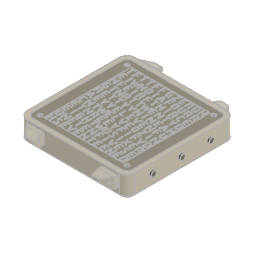
Wordy Watch v19 (Autodesk Fusion 360 design; units mm, degrees)
Autodesk Fusion 360 part; units mm, degrees
(part 1 of 4)
sketch "BatteryProfile" plane through (0, 0, 0) normal (0, 1, 0) x (1, 0, 0) in component "LiPo Battery"
  line L0 (-8.25, -1.75) -> (8.25, -1.75)
  line L1 (0, 0) -> (0, -1.75) construction
  line L2 (0, 0) -> (1, 0) construction
  line L3 (-8.25, 1.75) -> (8.25, 1.75)
  arc A0 (-8.25, 1.75) -> (-8.25, -1.75) centre (-8.25, 0) ccw
  arc A1 (8.25, -1.75) -> (8.25, 1.75) centre (8.25, 0) ccw
  line L4 (8.25, -1.75) -> (8.25, 1.75) construction
  line L5 (-8.25, -1.75) -> (-8.25, 1.75) construction
  point P0 (0, -1.75)
  dimension "d4" = 16.5
  dimension "d7" = 1.75
  dimension "d8" = 1
  constraint horizontal L0
  constraint coincident L1.start L2.start
  constraint vertical L1
  constraint midpoint L0 P0
  constraint coincident P0 L1.end
  constraint perpendicular L1 L2
  constraint symmetric L0.start L2 L3.start
  constraint symmetric L0.end L2 L3.end
  constraint coincident A1.centre L4
  constraint coincident A0.centre L5
  measures "d4" distance of L0.start L0.end
  measures "d7" distance of L1.start P0
  measures "d8" distance of L1.start L2.end
extrude "Extrude1" add sketch "BatteryProfile" along normal blind 25 makes body 1 in component "LiPo Battery"
sketch "PCBTop" plane through (0, 0, 0) normal (0, 0, 1) x (1, 0, 0) in component "PCB"
  line L0 (18, -18) -> (-18, -18)
  line L1 (-18, -18) -> (-18, 18)
  line L2 (-18, 18) -> (18, 18)
  line L3 (18, 18) -> (18, -18)
  line L4 (18, -18) -> (-18, 18) construction
  line L5 (-18, -18) -> (18, 18) construction
  line L6 (-9, -7.5) -> (-17, -7.5)
  line L7 (-17, -7.5) -> (-17, -13)
  line L8 (-17, -13) -> (-9, -13)
  line L9 (-9, -13) -> (-9, -7.5)
  line L10 (-9, -7.5) -> (-17, -13) construction
  line L11 (-17, -7.5) -> (-9, -13) construction
  line L12 (17.5, 8.6) -> (14.5, 8.6)
  line L13 (14.5, 8.6) -> (14.5, 13.4)
  line L14 (14.5, 13.4) -> (17.5, 13.4)
  line L15 (17.5, 13.4) -> (17.5, 8.6)
  line L16 (17.5, 8.6) -> (14.5, 13.4) construction
  line L17 (14.5, 8.6) -> (17.5, 13.4) construction
  line L18 (17.5, -2.4) -> (14.5, -2.4)
  line L19 (14.5, -2.4) -> (14.5, 2.4)
  line L20 (14.5, 2.4) -> (17.5, 2.4)
  line L21 (17.5, 2.4) -> (17.5, -2.4)
  line L22 (17.5, -13.4) -> (14.5, -13.4)
  line L23 (14.5, -13.4) -> (14.5, -8.6)
  line L24 (14.5, -8.6) -> (17.5, -8.6)
  line L25 (17.5, -8.6) -> (17.5, -13.4)
  line L26 (16.5, -16.5) -> (-16.5, -16.5) construction
  line L27 (-16.5, -16.5) -> (-16.5, 16.5) construction
  line L28 (-16.5, 16.5) -> (16.5, 16.5) construction
  line L29 (16.5, 16.5) -> (16.5, -16.5) construction
  line L30 (16.5, -16.5) -> (-16.5, 16.5) construction
  line L31 (-16.5, -16.5) -> (16.5, 16.5) construction
  circle A0 centre (-16.5, 16.5) radius 0.8
  circle A1 centre (16.5, 16.5) radius 0.8
  circle A2 centre (16.5, -16.5) radius 0.8
  circle A3 centre (-16.5, -16.5) radius 0.8
  point P0 (-13, -10.25)
  point P1 (16, 11)
  dimension "d79" = 36
  dimension "d80" = 36
  dimension "d83" = 8
  dimension "d84" = 5.5
  dimension "d85" = 5
  dimension "d87" = 3
  dimension "d88" = 4.8
  dimension "d89" = 2
  dimension "d90" = 7
  dimension "d93" = 11
  dimension "d94" = -22
  dimension "d178" = 33
  dimension "d179" = 33
  dimension "d180" = 1.6
  dimension "d181" = 1.6
  dimension "d182" = 1.6
  dimension "d183" = 1.6
  dimension "d239" = 7.75
  constraint horizontal L0
  constraint perpendicular L0 L1
  constraint parallel L0 L2
  constraint parallel L1 L3
  constraint coincident L4 origin
  constraint coincident L5 origin
  constraint horizontal L6
  constraint perpendicular L6 L7
  constraint parallel L6 L8
  constraint parallel L7 L9
  constraint coincident L10 P0
  constraint coincident L11 P0
  constraint horizontal L12
  constraint perpendicular L12 L13
  constraint parallel L12 L14
  constraint parallel L13 L15
  constraint coincident L16 P1
  constraint coincident L17 P1
  constraint horizontal L26
  constraint perpendicular L26 L27
  constraint parallel L26 L28
  constraint parallel L27 L29
  constraint coincident L30 origin
  constraint coincident L31 origin
  constraint coincident L27.end L28.start
  constraint coincident L28.end L29.start
  constraint coincident L26.start L29.end
  constraint coincident L26.end L27.start
  measures "d79" distance of L1.end L2.end
  measures "d80" distance of L0.end L1.end
  measures "d83" distance of L7.end L8.end
  measures "d84" distance of L6.end L7.end
  measures "d85" distance of L1 P0
  measures "d87" distance of L13.end L14.end
  measures "d88" distance of L12.end L13.end
  measures "d89" distance of L3 P1
  measures "d90" distance of L2 P1
  measures "d178" distance of L27.end L28.end
  measures "d179" distance of L26.end L27.end
  measures "d180" diameter of A0
  measures "d181" diameter of A1
  measures "d182" diameter of A2
  measures "d183" diameter of A3
  measures "d239" distance of L0 P0
sketch "USBC" plane through (0, 0, 0) normal (1, 0, 0) x (0, 1, 0) in component "PCB"
  line L0 (-18, 0) -> (18, 0)
  line L1 (4.1, 1) -> (9.9, 1)
  line L2 (9.9, 1) -> (9.9, 3.7)
  line L3 (9.9, 3.7) -> (4.1, 3.7)
  line L4 (4.1, 3.7) -> (4.1, 1)
  line L5 (4.1, 1) -> (9.9, 3.7) construction
  line L6 (9.9, 1) -> (4.1, 3.7) construction
  arc A0 (4.1, 3.7) -> (4.1, 1) centre (4.1, 2.35) ccw
  arc A1 (9.9, 1) -> (9.9, 3.7) centre (9.9, 2.35) ccw
  line L7 (7, 1) -> (7, 0) construction
  line L8 (4.1, 1) -> (4.1, 0)
  line L9 (9.9, 1) -> (9.9, 0)
  line L10 (9.9, 0) -> (4.1, 0)
  point P0 (7, 2.35)
  point P1 (7, 3.7)
  point P2 (18, 0)
  dimension "d95" = 5.8
  dimension "d96" = 2.7
  dimension "d103" = 1
  dimension "d238" = 11
  constraint horizontal L1
  constraint perpendicular L1 L2
  constraint parallel L1 L3
  constraint parallel L2 L4
  constraint coincident L5 P0
  constraint coincident L6 P0
  constraint midpoint L4 A0.centre
  constraint midpoint L2 A1.centre
  constraint midpoint L3 P1
  constraint midpoint L1 L7.start
  constraint coincident L0 L7.end
  constraint perpendicular L0 L7
  constraint coincident L0 L8.end
  constraint perpendicular L0 L8
  constraint coincident L0 L9.end
  constraint perpendicular L0 L9
  measures "d95" distance of L2.end L3.end
  measures "d96" distance of L1.end L2.end
  measures "d103" distance of L0 L1
  measures "d238" distance of L7.end P2
extrude "Extrude1'" add sketch "PCBTop" along normal blind 0.8 separate body contours L0 L1 L2 L3 | L6 L7 L8 L9 | L12 L13 L14 L15 | L18 L19 L20 L21 | L22 L23 L24 L25 makes body 2 in component "PCB"
extrude "Extrude2" add sketch "PCBTop" along normal blind 2.8 contours L12 L13 L14 L15 | L18 L19 L20 L21 | L22 L23 L24 L25 bodies 2 in component "PCB"
extrude "Extrude3" add sketch "PCBTop" along normal blind 3.8 contours L6 L7 L8 L9 bodies 2 in component "PCB"
extrude "Extrude4" add sketch "USBC" along normal blind 7 and the other way blind 1 from surface at -18 bodies 2 in component "PCB"
fillet "Fillet1" radius 2 4 edges at (-18, -18, 0.4) (18, -18, 0.4) (18, 18, 0.4) (-18, 18, 0.4) on bodies 2 in component "PCB"
sketch "ButtonBack" plane through (0, 0, 0) normal (0, 0, 1) x (1, 0, 0) in component "Case Button"
  line L0 (1.1, -0.55) -> (-1.1, -0.55)
  line L1 (-1.1, -0.55) -> (-1.1, 0.55)
  line L2 (-1.1, 0.55) -> (1.1, 0.55)
  line L3 (1.1, 0.55) -> (1.1, -0.55)
  line L4 (1.1, -0.55) -> (-1.1, 0.55) construction
  line L5 (-1.1, -0.55) -> (1.1, 0.55) construction
  circle A0 centre (0, 0) radius 1.75
  line L6 (-1.1, 0.55) -> (-1.1, 1.3611)
  line L7 (1.1, 0.55) -> (1.1, 1.3611)
  dimension "d202" = 1.1
  dimension "d203" = 2.2
  dimension "d204" = 3.5
  constraint horizontal L0
  constraint perpendicular L0 L1
  constraint parallel L0 L2
  constraint parallel L1 L3
  constraint coincident L4 A0.centre
  constraint coincident L5 A0.centre
  constraint coincident A0.centre origin
  constraint coincident A0 L6.end
  constraint perpendicular L2 L6
  constraint coincident A0 L7.end
  constraint perpendicular L2 L7
  measures "d202" distance of L0.end L1.end
  measures "d203" distance of L1.end L2.end
  measures "d204" diameter of A0
sketch "ButtonFront" plane through (0, 0, 0) normal (0, 0, 1) x (1, 0, 0) in component "Case Button"
  circle A0 centre (0, 0) radius 1
  dimension "d205" = 2
  constraint coincident A0.centre origin
  measures "d205" diameter of A0
extrude "Extrude1''" add sketch "ButtonBack" along normal blind 0.5 separate body contours L0 L1 L3 A0 L6 L7 makes body 3 in component "Case Button"
extrude "Extrude2'" add sketch "ButtonBack" along normal blind 0.5 from surface at 0.5 bodies 3 in component "Case Button"
extrude "Extrude3'" add sketch "ButtonFront" along normal blind 1.6 from surface at 1 bodies 3 in component "Case Button"
pattern_linear "R-Pattern1" count 3 spacing 11 along (1, 0, 0) of bodies 3 makes body 4 at (11.9988, -0.0498, 2.0667) makes body 5 at (22.9988, -0.0498, 2.0667) in component "Case Button"
sketch "CaseOuter" plane through (0, 0, 0) normal (0, 0, 1) x (1, 0, 0) in component "WatchCase"
  line L0 (-20.5, 20.5) -> (20.5, 20.5)
  line L1 (20.5, 20.5) -> (20.5, -20.5)
  line L2 (20.5, -20.5) -> (-20.5, -20.5)
  line L3 (-20.5, -20.5) -> (-20.5, 20.5)
  line L4 (-20.5, 20.5) -> (20.5, -20.5) construction
  line L5 (20.5, 20.5) -> (-20.5, -20.5) construction
  line L6 (-18.9, -18.9) -> (-18.9, 18.9)
  line L7 (-18.9, 18.9) -> (18.9, 18.9)
  line L8 (18.9, 18.9) -> (18.9, -18.9)
  line L9 (18.9, -18.9) -> (-18.9, -18.9)
  dimension "d42" = 41
  dimension "d43" = 41
  dimension "d44" = 1.6
  constraint horizontal L0
  constraint perpendicular L0 L1
  constraint parallel L0 L2
  constraint parallel L1 L3
  constraint coincident L4 origin
  constraint coincident L5 origin
  measures "d42" distance of L1.end L2.end
  measures "d43" distance of L0.end L1.end
sketch "CaseFixing" plane through (0, 0, 0) normal (0, 0, 1) x (1, 0, 0) in component "WatchCase"
  line L0 (16.5, -16.5) -> (-16.5, -16.5) construction
  line L1 (-16.5, -16.5) -> (-16.5, 16.5) construction
  line L2 (-16.5, 16.5) -> (16.5, 16.5) construction
  line L3 (16.5, 16.5) -> (16.5, -16.5) construction
  line L4 (16.5, -16.5) -> (-16.5, 16.5) construction
  line L5 (-16.5, -16.5) -> (16.5, 16.5) construction
  circle A0 centre (-16.5, 16.5) radius 0.6
  circle A1 centre (16.5, 16.5) radius 0.6
  circle A2 centre (-16.5, -16.5) radius 0.6
  circle A3 centre (16.5, -16.5) radius 0.6
  dimension "d32" = 33
  dimension "d33" = 33
  dimension "d34" = 1.2
  dimension "d35" = 1.2
  dimension "d36" = 1.2
  dimension "d37" = 1.2
  constraint horizontal L0
  constraint perpendicular L0 L1
  constraint parallel L0 L2
  constraint parallel L1 L3
  constraint coincident L4 origin
  constraint coincident L5 origin
  constraint coincident L1.end L2.start
  constraint coincident L2.end L3.start
  constraint coincident L0.end L1.start
  constraint coincident L0.start L3.end
  measures "d32" distance of L0.end L1.end
  measures "d33" distance of L1.end L2.end
  measures "d34" diameter of A0
  measures "d35" diameter of A1
  measures "d36" diameter of A2
  measures "d37" diameter of A3
sketch "CaseFixingBoss" plane through (0, 0, 0) normal (0, 0, 1) x (1, 0, 0) in component "WatchCase"
  line L0 (16.5, 16.5) -> (16.5, -16.5) construction
  circle A0 centre (-16.5, 16.5) radius 2.3
  circle A1 centre (16.5, 16.5) radius 2.3
  circle A2 centre (-16.5, -16.5) radius 2.3
  circle A3 centre (16.5, -16.5) radius 2.3
  line L1 (-16.5, 16.5) -> (16.5, 16.5) construction
  line L2 (-16.5, -16.5) -> (-16.5, 16.5) construction
  line L3 (16.5, -16.5) -> (-16.5, -16.5) construction
  dimension "d38" = 4.6
  dimension "d39" = 4.6
  dimension "d40" = 4.6
  dimension "d41" = 4.6
  constraint coincident A0.centre L1.start
  constraint coincident L0.start A1.centre
  constraint coincident A2.centre L2.start
  constraint coincident L0.end A3.centre
  measures "d38" diameter of A0
  measures "d39" diameter of A1
  measures "d40" diameter of A2
  measures "d41" diameter of A3
extrude "Extrude1'''" add sketch "CaseOuter" along normal blind 1.3 separate body contours L0 L1 L2 L3 | L6 L7 L8 L9 makes body 6 in component "WatchCase"
sketch "CaseCorners" plane through (0, 0, 0) normal (0, 0, 1) x (1, 0, 0) in component "WatchCase"
  line L0 (-20.5, -20.5) -> (20.5, -20.5)
  line L1 (20.5, -20.5) -> (20.5, 20.5)
  line L2 (20.5, 20.5) -> (-20.5, 20.5)
  line L3 (-20.5, 20.5) -> (-20.5, -20.5)
  line L4 (-16.5, 16.5) -> (16.5, 16.5)
  line L5 (-16.5, -16.5) -> (-16.5, 16.5)
  line L6 (16.5, -16.5) -> (-16.5, -16.5)
  line L7 (16.5, 16.5) -> (16.5, -16.5)
  line L8 (-16.5, 16.5) -> (-16.5, 20.5)
  line L9 (-16.5, 16.5) -> (-20.5, 16.5)
  line L10 (16.5, 16.5) -> (16.5, 20.5)
  line L11 (16.5, 16.5) -> (20.5, 16.5)
  line L12 (16.5, -16.5) -> (16.5, -20.5)
  line L13 (16.5, -16.5) -> (20.5, -16.5)
  line L14 (-16.5, -16.5) -> (-16.5, -20.5)
  line L15 (-16.5, -16.5) -> (-20.5, -16.5)
  constraint coincident L4.start L5.end
  constraint coincident L2 L8.end
  constraint perpendicular L2 L8
  constraint coincident L3 L9.end
  constraint perpendicular L3 L9
  constraint coincident L4.end L7.start
  constraint coincident L2 L10.end
  constraint perpendicular L2 L10
  constraint coincident L1 L11.end
  constraint perpendicular L1 L11
  constraint coincident L6.start L7.end
  constraint coincident L0 L12.end
  constraint perpendicular L0 L12
  constraint coincident L1 L13.end
  constraint perpendicular L1 L13
  constraint coincident L5.start L6.end
  constraint coincident L0 L14.end
  constraint perpendicular L0 L14
  constraint coincident L3 L15.end
  constraint perpendicular L3 L15
extrude "Extrude2''" add sketch "CaseFixingBoss" along normal blind 4.5 from surface at 1.3 separate body makes body 7 at (18.7971, 16.3854, 4.3) makes body 8 at (18.7971, -16.6146, 4.3) makes body 9 at (-14.2029, 16.3854, 4.3) makes body 10 at (-14.2029, -16.6146, 4.3) in component "WatchCase"
extrude "Extrude3''" add sketch "CaseOuter" along normal blind 8.1 bodies 6 in component "WatchCase"
extrude "Extrude4'" add sketch "CaseCorners" along normal up to surface (5.8 mm away) contours L0 L3 L14 L15 | L0 L1 L12 L13 | L2 L3 L8 L9 | L1 L2 L10 L11 bodies 6 7 8 9 10 in component "WatchCase"
extrude "Extrude5" cut sketch "CaseFixing" along normal up to surface (4.8 mm away) from surface at 1 bodies 6 in component "WatchCase"
fillet "Fillet1'" radius 2 4 edges at (18.9, 18.9, 6.95) (-18.9, 18.9, 6.95) (18.9, -18.9, 6.95) (-18.9, -18.9, 6.95) on bodies 6 in component "WatchCase"
fillet "Fillet2" radius 3 4 edges at (20.5, -20.5, 4.05) (-20.5, -20.5, 4.05) (-20.5, 20.5, 4.05) (20.5, 20.5, 4.05) on bodies 6 in component "WatchCase"
chamfer "Chamfer1" distance 1 angle 45 8 edges at (0, -20.5, 0) (-19.6213, -19.6213, 0) (-20.5, 0, 0) (-19.6213, 19.6213, 0) (0, 20.5, 0) (19.6213, 19.6213, 0) (20.5, 0, 0) (19.6213, -19.6213, 0) on bodies 6 in component "WatchCase"
sketch "Strap Bracket" plane through (0, 0, 0) normal (0, 0, 1) x (1, 0, 0) in component "WatchCase"
  line L0 (17.5, 20.5) -> (-17.5, 20.5)
  line L1 (-17.5, -20.5) -> (17.5, -20.5)
  line L2 (-17, 24.5) -> (-11, 24.5)
  line L3 (-11, 24.5) -> (-11, 20.5)
  line L4 (-11, 20.5) -> (-17, 20.5)
  line L5 (-17, 20.5) -> (-17, 24.5)
  line L6 (11, 24.5) -> (17, 24.5)
  line L7 (17, 24.5) -> (17, 20.5)
  line L8 (17, 20.5) -> (11, 20.5)
  line L9 (11, 20.5) -> (11, 24.5)
  line L10 (17.5, 20.5) -> (17.5, -20.5) construction
  line L11 (17.5, 0) -> (12.5, 0) construction
  point P0 (0, 20.5)
  dimension "d149" = 6
  dimension "d150" = 4
  dimension "d151" = 6
  dimension "d152" = 4
  dimension "d153" = 11
  dimension "d154" = 11
  dimension "d155" = 5
  constraint horizontal L2
  constraint vertical L3
  constraint horizontal L4
  constraint vertical L5
  constraint midpoint L0 P0
  constraint coincident L0 L3.end
  constraint horizontal L6
  constraint vertical L7
  constraint horizontal L8
  constraint vertical L9
  constraint coincident L0 L8.end
  constraint coincident L0.start L10.start
  constraint coincident L1.end L10.end
  constraint midpoint L10 L11.start
  constraint perpendicular L10 L11
  measures "d149" distance of L2.start L2.end
  measures "d150" distance of L2.start L4.end
  measures "d151" distance of L6.start L6.end
  measures "d152" distance of L6.start L8.end
  measures "d153" distance of L3.end P0
  measures "d154" distance of P0 L8.end
  measures "d155" distance of L11.start L11.end
extrude "Extrude6" add sketch "Strap Bracket" against normal blind 4 from surface at 7.1 separate body makes body 11 at (-13, 20.5, 4.4333) makes body 12 at (13, 24.5, 5.7667) in component "WatchCase"
sketch "BracketProfile" plane through (17, 0, 0) normal (1, 0, 0) x (0, 1, 0) in component "WatchCase"
  line L0 (24.5, 7.1) -> (20.5, 7.1)
  line L1 (20.5, 3.1) -> (24.5, 3.1)
  line L2 (24.5, 3.1) -> (24.5, 7.1)
  line L3 (20.5, 7.1) -> (24.5, 3.1) construction
  circle A0 centre (22.5, 5.1) radius 0.5
  line L4 (20.5, 7.1) -> (20.5, 3.1)
  dimension "d162" = 1
  constraint coincident L0.end L3.start
  constraint coincident L1.end L2.start
  constraint midpoint L3 A0.centre
  measures "d162" diameter of A0
extrude "Extrude7" cut sketch "BracketProfile" against normal blind 10 from surface at -28 contours A0 bodies 12 6 11 in component "WatchCase"
extrude "Extrude8" cut sketch "BracketProfile" along normal blind 10 from surface at -6 contours A0 bodies 12 11 6 in component "WatchCase"
chamfer "Chamfer2" distance 1 angle 70 2 edges at (14, 24.5, 7.1) (-14, 24.5, 7.1) measured on face at (13, 24.5, 5.7667) measured on face at (-15, 24.5, 5.7667) on bodies 11 12 in component "WatchCase"
chamfer "Chamfer3" distance 2 angle 45 2 edges at (14, 24.5, 3.1) (-14, 24.5, 3.1) measured on face at (13, 23.1667, 3.1) measured on face at (-13, 21.8333, 3.1) on bodies 11 12 in component "WatchCase"
chamfer "Chamfer4" distance 3 angle 45 2 edges at (17, 24.5, 5.6) (-17, 24.5, 5.6) measured on face at (13, 24.5, 5.7667) measured on face at (-17, 21, 5.1) on bodies 11 12 in component "WatchCase"
mirror "Mirror1" about plane through (0, 0, 0) normal (0, 1, 0) of bodies 12 11 makes body 13 at (-13, -20.5, 4.4333) makes body 14 at (15, -20.5, 5.7667) in component "WatchCase"
combine "Combine1" operation add target body 6 tool bodies 11 12 14 13 in component "WatchCase"
sketch "USBC (2)" plane through (-20.5, 0, 0) normal (-1, 0, 0) x (0, -1, 0) in component "WatchCase"
  line L0 (-17.5, 1) -> (17.5, 1)
  line L1 (17.5, 1) -> (17.5, 8.1)
  line L2 (17.5, 8.1) -> (-17.5, 8.1)
  line L3 (-17.5, 8.1) -> (-17.5, 1)
  line L4 (4.1, 2.9) -> (9.9, 2.9)
  arc A0 (9.9, 2.9) -> (9.9, 5.6) centre (9.9, 4.25) ccw
  line L5 (9.9, 5.6) -> (9.9, 6.6)
  line L6 (9.9, 6.6) -> (4.1, 6.6)
  line L7 (4.1, 6.6) -> (4.1, 5.6)
  arc A1 (4.1, 5.6) -> (4.1, 2.9) centre (4.1, 4.25) ccw
  line L8 (10.1, 6.8) -> (3.9, 6.8)
  line L9 (3.9, 6.8) -> (3.9, 5.787)
  arc A2 (3.9, 5.787) -> (4.1, 2.7) centre (4.1, 4.25) ccw
  line L10 (4.1, 2.7) -> (9.9, 2.7)
  arc A3 (9.9, 2.7) -> (10.1, 5.787) centre (9.9, 4.25) ccw
  line L11 (10.1, 5.787) -> (10.1, 6.8)
  line L12 (3.9, 5.787) -> (10.1, 5.787)
  dimension "d184" = 0.2
extrude "Extrude9" cut sketch "USBC (2)" against normal up to surface (1.6 mm away) contours L4 A0 L5 L7 A1 L12 | L4 A0 L5 L7 A1 A2 L10 A3 L12 bodies 6 in component "WatchCase"
extrude "Extrude5'" cut sketch "USBC (2)" against normal up to surface (1.6 mm away) contours L4 A0 L5 L7 A1 L12 | L4 A0 L5 L7 A1 A2 L10 A3 L12 sketch seen with x (1, 0, 0) y (0, -1, 0) z (0, 0, -1) at (0, 0, 6.6) bodies 2 in component "PCB"
sketch "Buttons" plane through (20.5, 0, 0) normal (1, 0, 0) x (0, 1, 0) in component "WatchCase"
  line L0 (-17.5, 1) -> (17.5, 1)
  line L1 (17.5, 1) -> (17.5, 8.1)
  line L2 (17.5, 8.1) -> (-17.5, 8.1)
  line L3 (-17.5, 8.1) -> (-17.5, 1)
  line L4 (-8.6, 5.8) -> (-13.4, 5.8)
  line L5 (-13.4, 5.8) -> (-13.4, 3.8)
  line L6 (-13.4, 3.8) -> (-8.6, 3.8)
  line L7 (-8.6, 3.8) -> (-8.6, 5.8)
  line L8 (2.4, 5.8) -> (-2.4, 5.8)
  line L9 (-2.4, 5.8) -> (-2.4, 3.8)
  line L10 (-2.4, 3.8) -> (2.4, 3.8)
  line L11 (2.4, 3.8) -> (2.4, 5.8)
  line L12 (13.4, 5.8) -> (8.6, 5.8)
  line L13 (8.6, 5.8) -> (8.6, 3.8)
  line L14 (8.6, 3.8) -> (13.4, 3.8)
  line L15 (13.4, 3.8) -> (13.4, 5.8)
  line L16 (-13.4, 5.8) -> (-8.6, 3.8) construction
  line L17 (-10.04, 4.4) -> (-11.96, 4.4)
  line L18 (-11.96, 4.4) -> (-11.96, 5.2)
  line L19 (-11.96, 5.2) -> (-10.04, 5.2)
  line L20 (-10.04, 5.2) -> (-10.04, 4.4)
  line L21 (-10.04, 4.4) -> (-11.96, 5.2) construction
  line L22 (-11.96, 4.4) -> (-10.04, 5.2) construction
  line L23 (0.96, 5.2) -> (0.96, 4.4)
  line L24 (0.96, 4.4) -> (-0.96, 4.4)
  line L25 (-0.96, 5.2) -> (0.96, 5.2)
  line L26 (-0.96, 4.4) -> (-0.96, 5.2)
  line L27 (11.96, 5.2) -> (11.96, 4.4)
  line L28 (10.04, 5.2) -> (11.96, 5.2)
  line L29 (10.04, 4.4) -> (10.04, 5.2)
  line L30 (11.96, 4.4) -> (10.04, 4.4)
  line L31 (-2.4, 5.8) -> (2.4, 3.8) construction
  line L32 (8.6, 5.8) -> (13.4, 3.8) construction
  line L33 (0.96, 5.2) -> (-0.96, 4.4) construction
  line L34 (11.96, 5.2) -> (10.04, 4.4) construction
  point P0 (-11, 4.8)
  point P1 (11, 4.8)
  point P2 (11, 4.8)
  point P3 (0, 4.8)
  point P4 (0, 4.8)
  dimension "d189" = 1.92
  dimension "d190" = 0.8
  dimension "d191" = 1.92
  dimension "d192" = 0.8
  dimension "d193" = 1.92
  dimension "d194" = 0.8
  constraint coincident L4.end L5.start
  constraint coincident L6.end L7.start
  constraint horizontal L17
  constraint perpendicular L17 L18
  constraint parallel L17 L19
  constraint parallel L18 L20
  constraint coincident L21 P0
  constraint coincident L22 P0
  constraint midpoint L16 P0
  constraint horizontal L24
  constraint perpendicular L24 L26
  constraint parallel L24 L25
  constraint parallel L23 L26
  constraint horizontal L30
  constraint perpendicular L29 L30
  constraint parallel L28 L30
  constraint parallel L27 L29
  constraint coincident L8.end L9.start
  constraint coincident L10.end L11.start
  constraint coincident L12.end L13.start
  constraint coincident L14.end L15.start
  constraint midpoint L34 P2
  constraint midpoint L32 P2
  constraint coincident P2 P1
  constraint midpoint L33 P4
  constraint midpoint L31 P4
  constraint coincident P4 P3
  measures "d189" distance of L18.end L19.end
  measures "d190" distance of L17.end L18.end
  measures "d191" distance of L25.start L23.start
  measures "d192" distance of L24.end L25.start
  measures "d193" distance of L28.start L27.start
  measures "d194" distance of L29.start L28.start
sketch "ButtonHoles" plane through (20.5, 0, 0) normal (1, 0, 0) x (0, 1, 0) in component "WatchCase"
  circle A0 centre (-11, 4.8) radius 1.2
  circle A1 centre (0, 4.8) radius 1.2
  circle A2 centre (11, 4.8) radius 1.2
  circle A3 centre (-11, 4.8) radius 1.95
  circle A4 centre (0, 4.8) radius 1.95
  circle A5 centre (11, 4.8) radius 1.95
  point P0 (-11, 4.8)
  point P1 (0, 4.8)
  point P2 (11, 4.8)
  dimension "d215" = 2.4
  dimension "d216" = 2.4
  dimension "d218" = 2.4
  dimension "d219" = 3.9
  dimension "d220" = 3.9
  dimension "d221" = 3.9
  constraint coincident P0 A0.centre
  constraint coincident P1 A1.centre
  constraint coincident P2 A2.centre
  constraint concentric A2 A5
  measures "d215" diameter of A0
  measures "d216" diameter of A1
  measures "d218" diameter of A2
  measures "d219" diameter of A3
  measures "d220" diameter of A4
  measures "d221" diameter of A5
extrude "Extrude6'" [suppressed] in component "PCB"
extrude "Extrude10" cut sketch "ButtonHoles" along normal blind 0.7 from surface at -1.6 contours A0 | A1 | A2 | A3 | A4 | A5 bodies 6 in component "WatchCase"
extrude "Extrude11" cut sketch "ButtonHoles" against normal up to surface (1.6 mm away) contours A0 | A1 | A2 bodies 6 in component "WatchCase"
sketch "Sketch1" plane through (0, 0, 0) normal (0, 0, 1) x (1, 0, 0) in component "Watch Face Text"
  line L0 (30.097, -17.6641) -> (60.097, -17.6641)
  line L1 (60.097, -17.6641) -> (60.097, 15.3359)
  line L2 (60.097, 15.3359) -> (30.097, 15.3359)
  line L3 (30.097, 15.3359) -> (30.097, -17.6641)
  line L4 (31.1779, 14.8177) -> (30.5921, 14.8605)
  line L5 (30.5921, 14.8605) -> (30.5702, 14.9689)
  line L6 (30.5702, 14.9689) -> (30.727, 15.0359)
  line L7 (30.727, 15.0359) -> (32.0867, 15.0041)
  line L8 (32.0867, 15.0041) -> (32.1306, 14.898)
  line L9 (32.1306, 14.898) -> (31.967, 14.8177)
  line L10 (31.967, 14.8177) -> (31.5161, 14.8177)
  line L11 (31.5161, 14.8177) -> (31.4941, 12.6904)
  line L12 (31.4941, 12.6904) -> (31.2624, 12.65)
  line L13 (31.2624, 12.65) -> (31.1779, 12.745)
  line L14 (31.1779, 12.745) -> (31.1779, 14.8177)
  line L15 (3.0809, 34.4818) -> (3.0809, 34.4818)
  line L16 (33.4792, 13.945) -> (34.3317, 13.9132)
  line L17 (34.3317, 13.9132) -> (34.3755, 13.8071)
  line L18 (34.3755, 13.8071) -> (34.2119, 13.7268)
  line L19 (34.2119, 13.7268) -> (33.4792, 13.7268)
  line L20 (33.4792, 13.7268) -> (33.4573, 12.6904)
  line L21 (33.4573, 12.6904) -> (33.2256, 12.65)
  line L22 (33.2256, 12.65) -> (33.141, 12.745)
  line L23 (33.141, 12.745) -> (33.1629, 14.9814)
  line L24 (33.1629, 14.9814) -> (33.3101, 15.0359)
  line L25 (33.3101, 15.0359) -> (34.5036, 15.0041)
  line L26 (34.5036, 15.0041) -> (34.5474, 14.8989)
  line L27 (34.5474, 14.8989) -> (34.3838, 14.8177)
  line L28 (34.3838, 14.8177) -> (33.4792, 14.8177)
  line L29 (33.4792, 14.8177) -> (33.4792, 13.945)
  line L30 (5.3822, 33.6091) -> (5.3822, 33.6091)
  line L31 (36.1779, 14.8177) -> (35.5921, 14.8605)
  line L32 (35.5921, 14.8605) -> (35.5702, 14.9689)
  line L33 (35.5702, 14.9689) -> (35.727, 15.0359)
  line L34 (35.727, 15.0359) -> (37.0867, 15.0041)
  line L35 (37.0867, 15.0041) -> (37.1306, 14.898)
  line L36 (37.1306, 14.898) -> (36.967, 14.8177)
  line L37 (36.967, 14.8177) -> (36.5161, 14.8177)
  line L38 (36.5161, 14.8177) -> (36.4941, 12.6904)
  line L39 (36.4941, 12.6904) -> (36.2624, 12.65)
  line L40 (36.2624, 12.65) -> (36.1779, 12.745)
  line L41 (36.1779, 12.745) -> (36.1779, 14.8177)
  line L42 (8.0809, 34.4818) -> (8.0809, 34.4818)
  line L43 (38.6779, 14.8177) -> (38.0921, 14.8605)
  line L44 (38.0921, 14.8605) -> (38.0702, 14.9689)
  line L45 (38.0702, 14.9689) -> (38.227, 15.0359)
  line L46 (38.227, 15.0359) -> (39.5867, 15.0041)
  line L47 (39.5867, 15.0041) -> (39.6306, 14.898)
  line L48 (39.6306, 14.898) -> (39.467, 14.8177)
  line L49 (39.467, 14.8177) -> (39.0161, 14.8177)
  line L50 (39.0161, 14.8177) -> (38.9941, 12.6904)
  line L51 (38.9941, 12.6904) -> (38.7624, 12.65)
  line L52 (38.7624, 12.65) -> (38.6779, 12.745)
  line L53 (38.6779, 12.745) -> (38.6779, 14.8177)
  line L54 (10.5809, 34.4818) -> (10.5809, 34.4818)
  line L55 (40.9792, 13.945) -> (41.8317, 13.9132)
  line L56 (41.8317, 13.9132) -> (41.8755, 13.8071)
  line L57 (41.8755, 13.8071) -> (41.7119, 13.7268)
  line L58 (41.7119, 13.7268) -> (40.9792, 13.7268)
  line L59 (40.9792, 13.7268) -> (40.9573, 12.6904)
  line L60 (40.9573, 12.6904) -> (40.7256, 12.65)
  line L61 (40.7256, 12.65) -> (40.641, 12.745)
  line L62 (40.641, 12.745) -> (40.6629, 14.9814)
  line L63 (40.6629, 14.9814) -> (40.8101, 15.0359)
  line L64 (40.8101, 15.0359) -> (42.0036, 15.0041)
  line L65 (42.0036, 15.0041) -> (42.0474, 14.8989)
  line L66 (42.0474, 14.8989) -> (41.8838, 14.8177)
  line L67 (41.8838, 14.8177) -> (40.9792, 14.8177)
  line L68 (40.9792, 14.8177) -> (40.9792, 13.945)
  line L69 (12.8822, 33.6091) -> (12.8822, 33.6091)
  line L70 (43.4792, 13.945) -> (44.3317, 13.9132)
  line L71 (44.3317, 13.9132) -> (44.3755, 13.8071)
  line L72 (44.3755, 13.8071) -> (44.2119, 13.7268)
  line L73 (44.2119, 13.7268) -> (43.4792, 13.7268)
  line L74 (43.4792, 13.7268) -> (43.4573, 12.6904)
  line L75 (43.4573, 12.6904) -> (43.2256, 12.65)
  line L76 (43.2256, 12.65) -> (43.141, 12.745)
  line L77 (43.141, 12.745) -> (43.1629, 14.9814)
  line L78 (43.1629, 14.9814) -> (43.3101, 15.0359)
  line L79 (43.3101, 15.0359) -> (44.5036, 15.0041)
  line L80 (44.5036, 15.0041) -> (44.5474, 14.8989)
  line L81 (44.5474, 14.8989) -> (44.3838, 14.8177)
  line L82 (44.3838, 14.8177) -> (43.4792, 14.8177)
  line L83 (43.4792, 14.8177) -> (43.4792, 13.945)
  line L84 (15.3822, 33.6091) -> (15.3822, 33.6091)
  line L85 (46.9045, 14.882) -> (46.9463, 14.7785)
  line L86 (46.9463, 14.7785) -> (46.7415, 14.703)
  line L87 (46.7415, 14.703) -> (46.4641, 14.8096)
  line L88 (46.4641, 14.8096) -> (46.1753, 14.7983)
  line L89 (46.1753, 14.7983) -> (45.9927, 14.7062)
  line L90 (45.9927, 14.7062) -> (45.9175, 14.608)
  line L91 (45.9175, 14.608) -> (45.9067, 13.0986)
  line L92 (45.9067, 13.0986) -> (45.9604, 12.9946)
  line L93 (45.9604, 12.9946) -> (46.1244, 12.8881)
  line L94 (46.1244, 12.8881) -> (46.347, 12.8507)
  line L95 (46.347, 12.8507) -> (46.7908, 12.8507)
  line L96 (46.7908, 12.8507) -> (46.7908, 13.6739)
  line L97 (46.7908, 13.6739) -> (46.4795, 13.7288)
  line L98 (46.4795, 13.7288) -> (46.4795, 13.835)
  line L99 (46.4795, 13.835) -> (46.6244, 13.8887)
  line L100 (46.6244, 13.8887) -> (47.091, 13.8466)
  line L101 (47.091, 13.8466) -> (47.1237, 13.7813)
  line L102 (47.1237, 13.7813) -> (47.1021, 12.6908)
  line L103 (47.1021, 12.6908) -> (46.9573, 12.6359)
  line L104 (46.9573, 12.6359) -> (46.2423, 12.64)
  line L105 (46.2423, 12.64) -> (45.9598, 12.7007)
  line L106 (45.9598, 12.7007) -> (45.7282, 12.8321)
  line L107 (45.7282, 12.8321) -> (45.6271, 12.9431)
  line L108 (45.6271, 12.9431) -> (45.5766, 13.0677)
  line L109 (45.5766, 13.0677) -> (45.5766, 14.6023)
  line L110 (45.5766, 14.6023) -> (45.6271, 14.7272)
  line L111 (45.6271, 14.7272) -> (45.7282, 14.8385)
  line L112 (45.7282, 14.8385) -> (45.9598, 14.9707)
  line L113 (45.9598, 14.9707) -> (46.2423, 15.0318)
  line L114 (46.2423, 15.0318) -> (46.5519, 15.0188)
  line L115 (46.5519, 15.0188) -> (46.9045, 14.882)
  line L116 (18.8076, 34.5461) -> (18.8076, 34.5461)
  line L117 (49.2471, 14.8177) -> (48.079, 14.8495)
  line L118 (48.079, 14.8495) -> (48.0352, 14.9556)
  line L119 (48.0352, 14.9556) -> (48.1988, 15.0359)
  line L120 (48.1988, 15.0359) -> (49.6149, 15.0041)
  line L121 (49.6149, 15.0041) -> (49.653, 14.885)
  line L122 (49.653, 14.885) -> (48.4468, 12.8541)
  line L123 (48.4468, 12.8541) -> (49.6149, 12.8223)
  line L124 (49.6149, 12.8223) -> (49.6588, 12.7171)
  line L125 (49.6588, 12.7171) -> (49.4951, 12.6359)
  line L126 (49.4951, 12.6359) -> (48.0818, 12.6686)
  line L127 (48.0818, 12.6686) -> (48.0466, 12.7941)
  line L128 (48.0466, 12.7941) -> (49.2471, 14.8177)
  line L129 (21.1502, 34.4818) -> (21.1502, 34.4818)
  line L130 (50.641, 12.745) -> (50.6629, 14.9814)
  line L131 (50.6629, 14.9814) -> (50.8101, 15.0359)
  line L132 (50.8101, 15.0359) -> (52.0036, 15.0041)
  line L133 (52.0036, 15.0041) -> (52.0474, 14.8989)
  line L134 (52.0474, 14.8989) -> (51.8838, 14.8177)
  line L135 (51.8838, 14.8177) -> (50.9792, 14.8177)
  line L136 (50.9792, 14.8177) -> (50.9792, 13.945)
  line L137 (50.9792, 13.945) -> (51.8317, 13.9132)
  line L138 (51.8317, 13.9132) -> (51.8755, 13.8071)
  line L139 (51.8755, 13.8071) -> (51.7119, 13.7268)
  line L140 (51.7119, 13.7268) -> (50.9792, 13.7268)
  line L141 (50.9792, 13.7268) -> (50.9792, 12.8541)
  line L142 (50.9792, 12.8541) -> (52.0036, 12.8223)
  line L143 (52.0036, 12.8223) -> (52.0474, 12.7171)
  line L144 (52.0474, 12.7171) -> (51.8838, 12.6359)
  line L145 (51.8838, 12.6359) -> (50.6903, 12.6677)
  line L146 (50.6903, 12.6677) -> (50.641, 12.745)
  line L147 (22.544, 32.4091) -> (22.544, 32.4091)
  line L148 (53.9963, 13.625) -> (54.1977, 13.7268)
  line L149 (54.1977, 13.7268) -> (54.2415, 13.8359)
  line L150 (54.2415, 13.8359) -> (54.2304, 14.6571)
  line L151 (54.2304, 14.6571) -> (54.1071, 14.7735)
  line L152 (54.1071, 14.7735) -> (53.9033, 14.8177)
  line L153 (53.9033, 14.8177) -> (53.3397, 14.8177)
  line L154 (53.3397, 14.8177) -> (53.3178, 12.6904)
  line L155 (53.3178, 12.6904) -> (53.0861, 12.65)
  line L156 (53.0861, 12.65) -> (53.0015, 12.745)
  line L157 (53.0015, 12.745) -> (53.0234, 14.9814)
  line L158 (53.0234, 14.9814) -> (53.1706, 15.0359)
  line L159 (53.1706, 15.0359) -> (54.0804, 15.0217)
  line L160 (54.0804, 15.0217) -> (54.3126, 14.9469)
  line L161 (54.3126, 14.9469) -> (54.4914, 14.8165)
  line L162 (54.4914, 14.8165) -> (54.5576, 14.7138)
  line L163 (54.5576, 14.7138) -> (54.5797, 14.5995)
  line L164 (54.5797, 14.5995) -> (54.5742, 13.7774)
  line L165 (54.5742, 13.7774) -> (54.5304, 13.6691)
  line L166 (54.5304, 13.6691) -> (54.2528, 13.4614)
  line L167 (54.2528, 13.4614) -> (54.684, 12.7123)
  line L168 (54.684, 12.7123) -> (54.4726, 12.6395)
  line L169 (54.4726, 12.6395) -> (54.3711, 12.6959)
  line L170 (54.3711, 12.6959) -> (53.8709, 13.5343)
  line L171 (53.8709, 13.5343) -> (53.9963, 13.625)
  line L172 (25.8994, 33.2891) -> (25.8994, 33.2891)
  line L173 (56.6117, 14.827) -> (56.5159, 14.9251)
  line L174 (56.5159, 14.9251) -> (56.6403, 15.0306)
  line L175 (56.6403, 15.0306) -> (56.9045, 14.9505)
  line L176 (56.9045, 14.9505) -> (57.0328, 14.8443)
  line L177 (57.0328, 14.8443) -> (57.1098, 14.7244)
  line L178 (57.1098, 14.7244) -> (57.1355, 14.5908)
  line L179 (57.1355, 14.5908) -> (57.129, 13.0125)
  line L180 (57.129, 13.0125) -> (57.0777, 12.8857)
  line L181 (57.0777, 12.8857) -> (56.9751, 12.7727)
  line L182 (56.9751, 12.7727) -> (56.662, 12.6368)
  line L183 (56.662, 12.6368) -> (56.5173, 12.7307)
  line L184 (56.5173, 12.7307) -> (56.7644, 12.9697)
  line L185 (56.7644, 12.9697) -> (56.7975, 13.081)
  line L186 (56.7975, 13.081) -> (56.7939, 14.6298)
  line L187 (56.7939, 14.6298) -> (56.7387, 14.7353)
  line L188 (56.7387, 14.7353) -> (56.6117, 14.827)
  line L189 (28.5147, 34.4911) -> (28.5147, 34.4911)
  line L190 (55.9105, 15.0159) -> (56.1561, 14.9802)
  line L191 (56.1561, 14.9802) -> (56.1567, 14.8728)
  line L192 (56.1567, 14.8728) -> (55.9552, 14.7353)
  line L193 (55.9552, 14.7353) -> (55.9001, 14.6298)
  line L194 (55.9001, 14.6298) -> (55.9001, 13.042)
  line L195 (55.9001, 13.042) -> (55.9552, 12.9365)
  line L196 (55.9552, 12.9365) -> (56.1766, 12.7615)
  line L197 (56.1766, 12.7615) -> (56.0916, 12.6518)
  line L198 (56.0916, 12.6518) -> (55.7894, 12.7213)
  line L199 (55.7894, 12.7213) -> (55.6611, 12.8275)
  line L200 (55.6611, 12.8275) -> (55.5841, 12.9474)
  line L201 (55.5841, 12.9474) -> (55.5585, 13.081)
  line L202 (55.5585, 13.081) -> (55.5649, 14.6593)
  line L203 (55.5649, 14.6593) -> (55.6162, 14.7861)
  line L204 (55.6162, 14.7861) -> (55.7188, 14.8991)
  line L205 (55.7188, 14.8991) -> (55.9105, 15.0159)
  line L206 (27.8135, 34.68) -> (27.8135, 34.68)
  line L207 (58.0029, 12.745) -> (58.0248, 14.9814)
  line L208 (58.0248, 14.9814) -> (58.2566, 15.0218)
  line L209 (58.2566, 15.0218) -> (58.3411, 14.9268)
  line L210 (58.3411, 14.9268) -> (58.3411, 13.945)
  line L211 (58.3411, 13.945) -> (59.3528, 13.945)
  line L212 (59.3528, 13.945) -> (59.3747, 14.9814)
  line L213 (59.3747, 14.9814) -> (59.6065, 15.0218)
  line L214 (59.6065, 15.0218) -> (59.691, 14.9268)
  line L215 (59.691, 14.9268) -> (59.6691, 12.6904)
  line L216 (59.6691, 12.6904) -> (59.4374, 12.65)
  line L217 (59.4374, 12.65) -> (59.3528, 12.745)
  line L218 (59.3528, 12.745) -> (59.3528, 13.7268)
  line L219 (59.3528, 13.7268) -> (58.3411, 13.7268)
  line L220 (58.3411, 13.7268) -> (58.3192, 12.6904)
  line L221 (58.3192, 12.6904) -> (58.0875, 12.65)
  line L222 (58.0875, 12.65) -> (58.0029, 12.745)
  line L223 (29.906, 32.4091) -> (29.906, 32.4091)
  line L224 (30.641, 9.745) -> (30.6629, 11.9814)
  line L225 (30.6629, 11.9814) -> (30.8101, 12.0359)
  line L226 (30.8101, 12.0359) -> (32.0036, 12.0041)
  line L227 (32.0036, 12.0041) -> (32.0474, 11.8989)
  line L228 (32.0474, 11.8989) -> (31.8838, 11.8177)
  line L229 (31.8838, 11.8177) -> (30.9792, 11.8177)
  line L230 (30.9792, 11.8177) -> (30.9792, 10.945)
  line L231 (30.9792, 10.945) -> (31.8317, 10.9132)
  line L232 (31.8317, 10.9132) -> (31.8755, 10.8071)
  line L233 (31.8755, 10.8071) -> (31.7119, 10.7268)
  line L234 (31.7119, 10.7268) -> (30.9792, 10.7268)
  line L235 (30.9792, 10.7268) -> (30.9792, 9.8541)
  line L236 (30.9792, 9.8541) -> (32.0036, 9.8223)
  line L237 (32.0036, 9.8223) -> (32.0474, 9.7171)
  line L238 (32.0474, 9.7171) -> (31.8838, 9.6359)
  line L239 (31.8838, 9.6359) -> (30.6903, 9.6677)
  line L240 (30.6903, 9.6677) -> (30.641, 9.745)
  line L241 (2.544, 29.4091) -> (2.544, 29.4091)
  line L242 (33.6779, 9.745) -> (33.6998, 11.9814)
  line L243 (33.6998, 11.9814) -> (33.9315, 12.0218)
  line L244 (33.9315, 12.0218) -> (34.0161, 11.9268)
  line L245 (34.0161, 11.9268) -> (33.9941, 9.6904)
  line L246 (33.9941, 9.6904) -> (33.7624, 9.65)
  line L247 (33.7624, 9.65) -> (33.6779, 9.745)
  line L248 (5.5809, 29.4091) -> (5.5809, 29.4091)
  line L249 (37.8536, 11.9032) -> (37.0749, 9.6686)
  line L250 (37.0749, 9.6686) -> (36.8768, 9.6586)
  line L251 (36.8768, 9.6586) -> (36.8187, 9.7304)
  line L252 (36.8187, 9.7304) -> (36.347, 11.105)
  line L253 (36.347, 11.105) -> (35.8321, 9.6686)
  line L254 (35.8321, 9.6686) -> (35.5775, 9.7191)
  line L255 (35.5775, 9.7191) -> (34.8489, 11.9689)
  line L256 (34.8489, 11.9689) -> (35.049, 12.0282)
  line L257 (35.049, 12.0282) -> (35.1422, 11.945)
  line L258 (35.1422, 11.945) -> (35.7256, 10.2123)
  line L259 (35.7256, 10.2123) -> (36.2442, 11.6432)
  line L260 (36.2442, 11.6432) -> (36.4535, 11.6414)
  line L261 (36.4535, 11.6414) -> (36.5093, 11.5632)
  line L262 (36.5093, 11.5632) -> (36.9684, 10.2123)
  line L263 (36.9684, 10.2123) -> (37.5974, 12.005)
  line L264 (37.5974, 12.005) -> (37.8117, 12.0041)
  line L265 (37.8117, 12.0041) -> (37.8536, 11.9032)
  line L266 (9.7566, 31.5673) -> (9.7566, 31.5673)
  line L267 (38.0029, 9.745) -> (38.0248, 11.9814)
  line L268 (38.0248, 11.9814) -> (38.2566, 12.0218)
  line L269 (38.2566, 12.0218) -> (38.3411, 11.9268)
  line L270 (38.3411, 11.9268) -> (38.3411, 10.945)
  line L271 (38.3411, 10.945) -> (39.3528, 10.945)
  line L272 (39.3528, 10.945) -> (39.3747, 11.9814)
  line L273 (39.3747, 11.9814) -> (39.6065, 12.0218)
  line L274 (39.6065, 12.0218) -> (39.691, 11.9268)
  line L275 (39.691, 11.9268) -> (39.6691, 9.6904)
  line L276 (39.6691, 9.6904) -> (39.4374, 9.65)
  line L277 (39.4374, 9.65) -> (39.3528, 9.745)
  line L278 (39.3528, 9.745) -> (39.3528, 10.7268)
  line L279 (39.3528, 10.7268) -> (38.3411, 10.7268)
  line L280 (38.3411, 10.7268) -> (38.3192, 9.6904)
  line L281 (38.3192, 9.6904) -> (38.0875, 9.65)
  line L282 (38.0875, 9.65) -> (38.0029, 9.745)
  line L283 (9.906, 29.4091) -> (9.906, 29.4091)
  line L284 (41.6117, 11.827) -> (41.5159, 11.9251)
  line L285 (41.5159, 11.9251) -> (41.6403, 12.0306)
  line L286 (41.6403, 12.0306) -> (41.9045, 11.9505)
  line L287 (41.9045, 11.9505) -> (42.0328, 11.8443)
  line L288 (42.0328, 11.8443) -> (42.1098, 11.7244)
  line L289 (42.1098, 11.7244) -> (42.1355, 11.5908)
  line L290 (42.1355, 11.5908) -> (42.129, 10.0125)
  line L291 (42.129, 10.0125) -> (42.0777, 9.8857)
  line L292 (42.0777, 9.8857) -> (41.9751, 9.7727)
  line L293 (41.9751, 9.7727) -> (41.662, 9.6368)
  line L294 (41.662, 9.6368) -> (41.5173, 9.7307)
  line L295 (41.5173, 9.7307) -> (41.7644, 9.9697)
  line L296 (41.7644, 9.9697) -> (41.7975, 10.081)
  line L297 (41.7975, 10.081) -> (41.7939, 11.6298)
  line L298 (41.7939, 11.6298) -> (41.7387, 11.7353)
  line L299 (41.7387, 11.7353) -> (41.6117, 11.827)
  line L300 (13.5147, 31.4911) -> (13.5147, 31.4911)
  line L301 (40.9105, 12.0159) -> (41.1561, 11.9802)
  line L302 (41.1561, 11.9802) -> (41.1567, 11.8728)
  line L303 (41.1567, 11.8728) -> (40.9552, 11.7353)
  line L304 (40.9552, 11.7353) -> (40.9001, 11.6298)
  line L305 (40.9001, 11.6298) -> (40.9001, 10.042)
  line L306 (40.9001, 10.042) -> (40.9552, 9.9365)
  line L307 (40.9552, 9.9365) -> (41.1766, 9.7615)
  line L308 (41.1766, 9.7615) -> (41.0916, 9.6518)
  line L309 (41.0916, 9.6518) -> (40.7894, 9.7213)
  line L310 (40.7894, 9.7213) -> (40.6611, 9.8275)
  line L311 (40.6611, 9.8275) -> (40.5841, 9.9474)
  line L312 (40.5841, 9.9474) -> (40.5585, 10.081)
  line L313 (40.5585, 10.081) -> (40.5649, 11.6593)
  line L314 (40.5649, 11.6593) -> (40.6162, 11.7861)
  line L315 (40.6162, 11.7861) -> (40.7188, 11.8991)
  line L316 (40.7188, 11.8991) -> (40.9105, 12.0159)
  line L317 (12.8135, 31.68) -> (12.8135, 31.68)
  line L318 (43.6779, 9.745) -> (43.6998, 11.9814)
  line L319 (43.6998, 11.9814) -> (43.9315, 12.0218)
  line L320 (43.9315, 12.0218) -> (44.0161, 11.9268)
  line L321 (44.0161, 11.9268) -> (43.9941, 9.6904)
  line L322 (43.9941, 9.6904) -> (43.7624, 9.65)
  line L323 (43.7624, 9.65) -> (43.6779, 9.745)
  line L324 (15.5809, 29.4091) -> (15.5809, 29.4091)
  line L325 (45.876, 10.3583) -> (46.4819, 10.3154)
  line L326 (46.4819, 10.3154) -> (46.5038, 10.207)
  line L327 (46.5038, 10.207) -> (46.347, 10.1399)
  line L328 (46.347, 10.1399) -> (45.7857, 10.1399)
  line L329 (45.7857, 10.1399) -> (45.5657, 9.6687)
  line L330 (45.5657, 9.6687) -> (45.3246, 9.6677)
  line L331 (45.3246, 9.6677) -> (45.2781, 9.7687)
  line L332 (45.2781, 9.7687) -> (46.2285, 12.0031)
  line L333 (46.2285, 12.0031) -> (46.4508, 12.0132)
  line L334 (46.4508, 12.0132) -> (46.5134, 11.9413)
  line L335 (46.5134, 11.9413) -> (47.4132, 9.7163)
  line L336 (47.4132, 9.7163) -> (47.2266, 9.6368)
  line L337 (47.2266, 9.6368) -> (47.0802, 9.7269)
  line L338 (47.0802, 9.7269) -> (46.347, 11.4991)
  line L339 (46.347, 11.4991) -> (45.876, 10.3583)
  line L340 (17.779, 30.0224) -> (17.779, 30.0224)
  line L341 (48.4792, 10.945) -> (49.3317, 10.9132)
  line L342 (49.3317, 10.9132) -> (49.3755, 10.8071)
  line L343 (49.3755, 10.8071) -> (49.2119, 10.7268)
  line L344 (49.2119, 10.7268) -> (48.4792, 10.7268)
  line L345 (48.4792, 10.7268) -> (48.4573, 9.6904)
  line L346 (48.4573, 9.6904) -> (48.2256, 9.65)
  line L347 (48.2256, 9.65) -> (48.141, 9.745)
  line L348 (48.141, 9.745) -> (48.1629, 11.9814)
  line L349 (48.1629, 11.9814) -> (48.3101, 12.0359)
  line L350 (48.3101, 12.0359) -> (49.5036, 12.0041)
  line L351 (49.5036, 12.0041) -> (49.5474, 11.8989)
  line L352 (49.5474, 11.8989) -> (49.3838, 11.8177)
  line L353 (49.3838, 11.8177) -> (48.4792, 11.8177)
  line L354 (48.4792, 11.8177) -> (48.4792, 10.945)
  line L355 (20.3822, 30.6091) -> (20.3822, 30.6091)
  line L356 (51.6117, 11.827) -> (51.5159, 11.9251)
  line L357 (51.5159, 11.9251) -> (51.6403, 12.0306)
  line L358 (51.6403, 12.0306) -> (51.9045, 11.9505)
  line L359 (51.9045, 11.9505) -> (52.0328, 11.8443)
  line L360 (52.0328, 11.8443) -> (52.1098, 11.7244)
  line L361 (52.1098, 11.7244) -> (52.1355, 11.5908)
  line L362 (52.1355, 11.5908) -> (52.129, 10.0125)
  line L363 (52.129, 10.0125) -> (52.0777, 9.8857)
  line L364 (52.0777, 9.8857) -> (51.9751, 9.7727)
  line L365 (51.9751, 9.7727) -> (51.662, 9.6368)
  line L366 (51.662, 9.6368) -> (51.5173, 9.7307)
  line L367 (51.5173, 9.7307) -> (51.7644, 9.9697)
  line L368 (51.7644, 9.9697) -> (51.7975, 10.081)
  line L369 (51.7975, 10.081) -> (51.7939, 11.6298)
  line L370 (51.7939, 11.6298) -> (51.7387, 11.7353)
  line L371 (51.7387, 11.7353) -> (51.6117, 11.827)
  line L372 (23.5147, 31.4911) -> (23.5147, 31.4911)
  line L373 (50.9105, 12.0159) -> (51.1561, 11.9802)
  line L374 (51.1561, 11.9802) -> (51.1567, 11.8728)
  line L375 (51.1567, 11.8728) -> (50.9552, 11.7353)
  line L376 (50.9552, 11.7353) -> (50.9001, 11.6298)
  line L377 (50.9001, 11.6298) -> (50.9001, 10.042)
  line L378 (50.9001, 10.042) -> (50.9552, 9.9365)
  line L379 (50.9552, 9.9365) -> (51.1766, 9.7615)
  line L380 (51.1766, 9.7615) -> (51.0916, 9.6518)
  line L381 (51.0916, 9.6518) -> (50.7894, 9.7213)
  line L382 (50.7894, 9.7213) -> (50.6611, 9.8275)
  line L383 (50.6611, 9.8275) -> (50.5841, 9.9474)
  line L384 (50.5841, 9.9474) -> (50.5585, 10.081)
  line L385 (50.5585, 10.081) -> (50.5649, 11.6593)
  line L386 (50.5649, 11.6593) -> (50.6162, 11.7861)
  line L387 (50.6162, 11.7861) -> (50.7188, 11.8991)
  line L388 (50.7188, 11.8991) -> (50.9105, 12.0159)
  line L389 (22.8135, 31.68) -> (22.8135, 31.68)
  line L390 (53.0691, 10.1378) -> (53.0907, 11.9821)
  line L391 (53.0907, 11.9821) -> (53.3191, 12.022)
  line L392 (53.3191, 12.022) -> (53.4025, 11.9284)
  line L393 (53.4025, 11.9284) -> (53.4061, 10.0993)
  line L394 (53.4061, 10.0993) -> (53.4605, 9.9952)
  line L395 (53.4605, 9.9952) -> (53.6259, 9.8884)
  line L396 (53.6259, 9.8884) -> (53.9066, 9.8533)
  line L397 (53.9066, 9.8533) -> (54.1159, 9.9095)
  line L398 (54.1159, 9.9095) -> (54.2588, 10.028)
  line L399 (54.2588, 10.028) -> (54.2915, 10.1378)
  line L400 (54.2915, 10.1378) -> (54.3131, 11.9821)
  line L401 (54.3131, 11.9821) -> (54.5415, 12.022)
  line L402 (54.5415, 12.022) -> (54.6249, 11.9284)
  line L403 (54.6249, 11.9284) -> (54.6185, 10.0702)
  line L404 (54.6185, 10.0702) -> (54.5679, 9.9451)
  line L405 (54.5679, 9.9451) -> (54.4667, 9.8336)
  line L406 (54.4667, 9.8336) -> (54.2347, 9.7012)
  line L407 (54.2347, 9.7012) -> (53.9518, 9.64)
  line L408 (53.9518, 9.64) -> (53.6426, 9.6522)
  line L409 (53.6426, 9.6522) -> (53.3754, 9.738)
  line L410 (53.3754, 9.738) -> (53.2273, 9.8336)
  line L411 (53.2273, 9.8336) -> (53.126, 9.9451)
  line L412 (53.126, 9.9451) -> (53.0691, 10.1378)
  line L413 (24.9721, 29.8019) -> (24.9721, 29.8019)
  line L414 (56.4963, 10.625) -> (56.6977, 10.7268)
  line L415 (56.6977, 10.7268) -> (56.7415, 10.8359)
  line L416 (56.7415, 10.8359) -> (56.7304, 11.6571)
  line L417 (56.7304, 11.6571) -> (56.6071, 11.7735)
  line L418 (56.6071, 11.7735) -> (56.4033, 11.8177)
  line L419 (56.4033, 11.8177) -> (55.8397, 11.8177)
  line L420 (55.8397, 11.8177) -> (55.8178, 9.6904)
  line L421 (55.8178, 9.6904) -> (55.5861, 9.65)
  line L422 (55.5861, 9.65) -> (55.5015, 9.745)
  line L423 (55.5015, 9.745) -> (55.5234, 11.9814)
  line L424 (55.5234, 11.9814) -> (55.6706, 12.0359)
  line L425 (55.6706, 12.0359) -> (56.5804, 12.0217)
  line L426 (56.5804, 12.0217) -> (56.8126, 11.9469)
  line L427 (56.8126, 11.9469) -> (56.9914, 11.8165)
  line L428 (56.9914, 11.8165) -> (57.0576, 11.7138)
  line L429 (57.0576, 11.7138) -> (57.0797, 11.5995)
  line L430 (57.0797, 11.5995) -> (57.0742, 10.7774)
  line L431 (57.0742, 10.7774) -> (57.0304, 10.6691)
  line L432 (57.0304, 10.6691) -> (56.7528, 10.4614)
  line L433 (56.7528, 10.4614) -> (57.184, 9.7123)
  line L434 (57.184, 9.7123) -> (56.9726, 9.6395)
  line L435 (56.9726, 9.6395) -> (56.8711, 9.6959)
  line L436 (56.8711, 9.6959) -> (56.3709, 10.5343)
  line L437 (56.3709, 10.5343) -> (56.4963, 10.625)
  line L438 (28.3994, 30.2891) -> (28.3994, 30.2891)
  line L439 (58.9963, 10.625) -> (59.1977, 10.7268)
  line L440 (59.1977, 10.7268) -> (59.2415, 10.8359)
  line L441 (59.2415, 10.8359) -> (59.2304, 11.6571)
  line L442 (59.2304, 11.6571) -> (59.1071, 11.7735)
  line L443 (59.1071, 11.7735) -> (58.9033, 11.8177)
  line L444 (58.9033, 11.8177) -> (58.3397, 11.8177)
  line L445 (58.3397, 11.8177) -> (58.3178, 9.6904)
  line L446 (58.3178, 9.6904) -> (58.0861, 9.65)
  line L447 (58.0861, 9.65) -> (58.0015, 9.745)
  line L448 (58.0015, 9.745) -> (58.0234, 11.9814)
  line L449 (58.0234, 11.9814) -> (58.1706, 12.0359)
  line L450 (58.1706, 12.0359) -> (59.0804, 12.0217)
  line L451 (59.0804, 12.0217) -> (59.3126, 11.9469)
  line L452 (59.3126, 11.9469) -> (59.4914, 11.8165)
  line L453 (59.4914, 11.8165) -> (59.5576, 11.7138)
  line L454 (59.5576, 11.7138) -> (59.5797, 11.5995)
  line L455 (59.5797, 11.5995) -> (59.5742, 10.7774)
  line L456 (59.5742, 10.7774) -> (59.5304, 10.6691)
  line L457 (59.5304, 10.6691) -> (59.2528, 10.4614)
  line L458 (59.2528, 10.4614) -> (59.684, 9.7123)
  line L459 (59.684, 9.7123) -> (59.4726, 9.6395)
  line L460 (59.4726, 9.6395) -> (59.3711, 9.6959)
  line L461 (59.3711, 9.6959) -> (58.8709, 10.5343)
  line L462 (58.8709, 10.5343) -> (58.9963, 10.625)
  line L463 (30.8994, 30.2891) -> (30.8994, 30.2891)
  line L464 (30.7274, 8.4473) -> (30.7055, 6.6904)
  line L465 (30.7055, 6.6904) -> (30.474, 6.65)
  line L466 (30.474, 6.65) -> (30.3895, 6.7449)
  line L467 (30.3895, 6.7449) -> (30.4114, 8.9814)
  line L468 (30.4114, 8.9814) -> (30.6436, 9.0222)
  line L469 (30.6436, 9.0222) -> (30.7077, 8.9796)
  line L470 (30.7077, 8.9796) -> (31.9665, 7.2336)
  line L471 (31.9665, 7.2336) -> (31.9884, 8.9814)
  line L472 (31.9884, 8.9814) -> (32.2199, 9.0218)
  line L473 (32.2199, 9.0218) -> (32.3044, 8.9269)
  line L474 (32.3044, 8.9269) -> (32.2831, 6.6906)
  line L475 (32.2831, 6.6906) -> (32.0516, 6.6504)
  line L476 (32.0516, 6.6504) -> (31.9749, 6.7086)
  line L477 (31.9749, 6.7086) -> (30.7274, 8.4473)
  line L478 (2.6305, 28.1114) -> (2.6305, 28.1114)
  line L479 (33.4792, 7.945) -> (34.3317, 7.9132)
  line L480 (34.3317, 7.9132) -> (34.3755, 7.8071)
  line L481 (34.3755, 7.8071) -> (34.2119, 7.7268)
  line L482 (34.2119, 7.7268) -> (33.4792, 7.7268)
  line L483 (33.4792, 7.7268) -> (33.4573, 6.6904)
  line L484 (33.4573, 6.6904) -> (33.2256, 6.65)
  line L485 (33.2256, 6.65) -> (33.141, 6.745)
  line L486 (33.141, 6.745) -> (33.1629, 8.9814)
  line L487 (33.1629, 8.9814) -> (33.3101, 9.0359)
  line L488 (33.3101, 9.0359) -> (34.5036, 9.0041)
  line L489 (34.5036, 9.0041) -> (34.5474, 8.8989)
  line L490 (34.5474, 8.8989) -> (34.3838, 8.8177)
  line L491 (34.3838, 8.8177) -> (33.4792, 8.8177)
  line L492 (33.4792, 8.8177) -> (33.4792, 7.945)
  line L493 (5.3822, 27.6091) -> (5.3822, 27.6091)
  line L494 (35.641, 6.745) -> (35.6629, 8.9814)
  line L495 (35.6629, 8.9814) -> (35.8101, 9.0359)
  line L496 (35.8101, 9.0359) -> (37.0036, 9.0041)
  line L497 (37.0036, 9.0041) -> (37.0474, 8.8989)
  line L498 (37.0474, 8.8989) -> (36.8838, 8.8177)
  line L499 (36.8838, 8.8177) -> (35.9792, 8.8177)
  line L500 (35.9792, 8.8177) -> (35.9792, 7.945)
  line L501 (35.9792, 7.945) -> (36.8317, 7.9132)
  line L502 (36.8317, 7.9132) -> (36.8755, 7.8071)
  line L503 (36.8755, 7.8071) -> (36.7119, 7.7268)